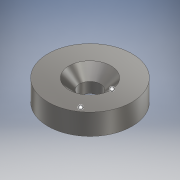
# Autodesk Inventor part: XY Metal Slug
Saved by Autodesk Inventor 2019 (Build 230136000, 136)
## iProperties
Created: 2018-10-20
Part Number: XY Metal Slug
Material: Steel, Carbon
Document SubType Name: Sheet Metal
Designer: Ax
Density: 7.85 g/cm^3
Sheet Metal Rule: Default_mm
Appearance: Semi-Polished
Mass: 11.0463 g
Surface Area: 9.66877 cm^2
Volume: 1.40717 cm^3
Author: Ax
Autodesk Inventor part; units mm, degrees
ref_plane "YZ Plane" through (0, 0, 0) normal (1, 0, 0) x (0, 1, 0)
ref_plane "XZ Plane" through (0, 0, 0) normal (0, 1, 0) x (-1, 0, 0)
ref_plane "XY Plane" through (0, 0, 0) normal (0, 0, 1) x (1, 0, 0)
sketch "Sketch1" plane through (0, 0, 0) normal (0, 0, 1) x (1, 0, 0)
  circle A0 centre (0, 0) radius 10
  dimension "d0" = 20
  measures "d0" diameter of A0
extrude "Plate1" add sketch "Sketch1" along normal blind 5
sketch "Sketch2" plane through (0, 0, 5) normal (0, 0, 1) x (1, 0, 0)
  circle A0 centre (0, 0) radius 1.204
  constraints: 1 centre point, 1 coincident
hole "Hole1" at (0, 0, 5) direction (0, 0, -1) diameter 5 end through all countersink diameter 10 countersink angle 90
equation "\"d8\" = Thickness"
equation "\"d2\" = Thickness"
equation "\"TransitionRadius\" = BendRadius"
equation "\"JacobiRadiusSize\" = BendRadius"
equation "\"d1\" = BendRadius"
equation "\"Thickness\" = 5"
equation "\"BendRadius\" = 0.8"
body "Solid1"
